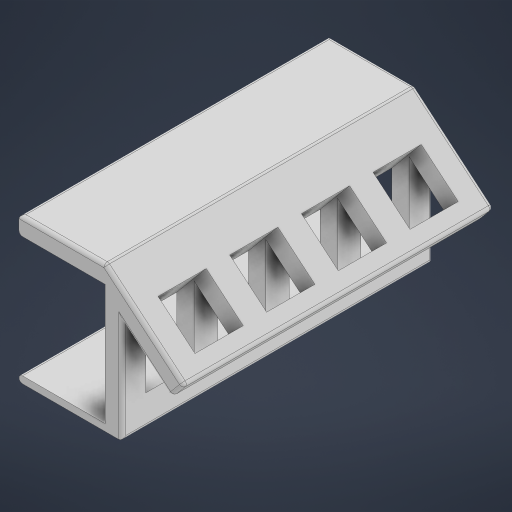
# Autodesk Inventor part: LightController-Case
Saved by Autodesk Inventor 2024 (Build 280153000, 153)
## iProperties
Created: 2024-09-09
Part Number: LightController-Case
Material: Generic
Document SubType Name: Modeling
Designer: Valentin
Density: 1 g/cm^3
Appearance: Default
Author: Valentin
Autodesk Inventor part; units mm, degrees
ref_plane "YZ Plane" through (0, 0, 0) normal (1, 0, 0) x (0, 1, 0)
ref_plane "XZ Plane" through (0, 0, 0) normal (0, 1, 0) x (-1, 0, 0)
ref_plane "XY Plane" through (0, 0, 0) normal (0, 0, 1) x (1, 0, 0)
sketch "Sketch1" plane through (0, 0, 0) normal (0, 1, 0) x (-1, 0, 0)
  line L0 (19.8276, 5.3853) -> (19.8276, -19.6147)
  line L1 (19.8276, -19.6147) -> (-15.1724, -19.6147)
  line L2 (-15.1724, -19.6147) -> (-15.1724, 5.3853)
  line L3 (19.8276, 5.3853) -> (24.8276, 5.3853)
  line L4 (24.8276, 5.3853) -> (24.8276, -19.6147)
  line L5 (24.8276, -19.6147) -> (19.8276, -19.6147)
  line L6 (19.8276, -19.6147) -> (19.8276, 5.3853)
  line L7 (24.8276, -19.6147) -> (5.544, -42.596)
  line L8 (24.8276, -19.6147) -> (54.8276, -19.6147) construction
  line L9 (5.544, -42.596) -> (0.9477, -38.7393)
  line L10 (0.9477, -38.7393) -> (16.9952, -19.6147)
  line L11 (-15.1724, -19.6147) -> (-15.1724, -24.6147)
  line L12 (-15.1724, -24.6147) -> (12.7997, -24.6147)
  line L13 (-15.1724, 5.3853) -> (-17.1724, 5.3853)
  line L14 (-17.1724, 5.3853) -> (-17.1724, -24.6147)
  line L15 (-17.1724, -24.6147) -> (-15.1724, -24.6147)
  point P0 (0, 0)
  dimension "d0" = 35
  dimension "d1" = 25
  dimension "d2" = 25
  dimension "d3" = 5
  dimension "d4" = 30
  dimension "d5" = 130
  dimension "d6" = 6
  dimension "d7" = 5
  dimension "d8" = 2
  constraints: 32 end point, 4 horizontal, 4 perpendicular, 3 vertical, 2 parallel, 2 point on line, 1 collinear, 1 equal length
  measures "d0" distance of L0.end L1.end
  measures "d1" distance of L1.end L2.end
  measures "d2" distance of L0.start L0.end
  measures "d3" distance of L4.end L5.end
  measures "d4" distance of L4.end L7.end
  measures "d5" angle of L7 L8
  measures "d6" distance of L7.end L9.end
  measures "d7" distance of L1.end L11.end
  measures "d8" distance of L2.end L13.end
extrude "Extrusion1" add sketch "Sketch1" along normal blind 90
sketch "Sketch2" plane through (-24.8276, 0, -19.6147) normal (-0.7660444, 0, -0.6427876) x (-0.6427876, 0, 0.7660444)
  line L0 (-25.1629, 83.2) -> (-11.1629, 83.2)
  line L1 (-11.1629, 83.2) -> (-11.1629, 69.2)
  line L2 (-11.1629, 69.2) -> (-25.1629, 69.2)
  line L3 (-25.1629, 69.2) -> (-25.1629, 83.2)
  line L4 (-25.1629, 62.4) -> (-11.1629, 62.4)
  line L5 (-11.1629, 62.4) -> (-11.1629, 48.4)
  line L6 (-11.1629, 48.4) -> (-25.1629, 48.4)
  line L7 (-25.1629, 48.4) -> (-25.1629, 62.4)
  line L8 (-11.1629, 41.6) -> (-11.1629, 27.6)
  line L9 (-25.1629, 41.6) -> (-11.1629, 41.6)
  line L10 (-25.1629, 27.6) -> (-25.1629, 41.6)
  line L11 (-11.1629, 27.6) -> (-25.1629, 27.6)
  line L12 (-11.1629, 20.8) -> (-11.1629, 6.8)
  line L13 (-25.1629, 20.8) -> (-11.1629, 20.8)
  line L14 (-25.1629, 6.8) -> (-25.1629, 20.8)
  line L15 (-11.1629, 6.8) -> (-25.1629, 6.8)
  line L16 (-25.7115, 90) -> (-6.5604, 90) projected
  point P0 (-0.9332, 0)
  dimension "d11" = 14
  dimension "d12" = 14
  dimension "d13" = 14
  dimension "d14" = 14
  dimension "d15" = 14
  dimension "d16" = 14
  dimension "d17" = 14
  dimension "d18" = 14
  dimension "d19" = 6.8
  dimension "d20" = 6.8
  dimension "d21" = 6.8
  dimension "d22" = 6.8
  constraints: 32 end point, 5 parallel, 4 horizontal, 4 perpendicular, 2 collinear
  measures "d11" distance of L1.end L2.end
  measures "d12" distance of L0.end L1.end
  measures "d13" distance of L5.end L7.start
  measures "d14" distance of L5.start L5.end
  measures "d15" distance of L8.end L10.start
  measures "d16" distance of L8.start L8.end
  measures "d17" distance of L12.end L14.start
  measures "d18" distance of L12.start L12.end
  measures "d19" distance between parallel lines of L16 L0
  measures "d20" distance between parallel lines of L4 L2
  measures "d21" distance between parallel lines of L9 L6
  measures "d22" distance between parallel lines of L13 L11
extrude "Extrusion2" cut sketch "Sketch2" against normal up to surface surface through (-19.8276, 0, -19.6147) normal (0, 0, 1)
move or copy body "Move Body1" bodies to move or copy 1 copy no rotation origin (0, 0, 0) rotation axis (-1, 0, 0) rotation angle -90 translate (0, -19.6147, -19.6147)
move or copy body "Move Body2" bodies to move or copy 1 copy no rotation origin (0, 0, 0) rotation axis (0, 0, 1) rotation angle -90 translate (12.1724, 22.1724, 0)
fillet "Fillet1" radius 1 18 edges at (-12.8276, 7, 25.3853) (-12.8276, 5, 25.3853) (17.1724, 5, 25.3853) (31.297, 23.1201, 25.3853) (35.1537, 27.7164, 25.3853) (33.2253, 25.4182, 70.3853) (24.2347, 29.0461, 70.3853) (23.663, 37.3582, 70.3853) (23.663, 37.3582, -19.6147) (33.2253, 25.4182, -19.6147) (24.2347, 29.0461, -19.6147) (17.1724, 19.986, -19.6147) (-0.3276, 47, -19.6147) (17.1724, 19.986, 70.3853) (-12.8276, 47, 25.3853) (-12.8276, 42, 25.3853) (-0.3276, 47, 70.3853) (12.1724, 47, 25.3853)
equation "\"d20\" = d19"
equation "\"d21\" = d19"
equation "\"d22\" = d19"
body "Solid1"
